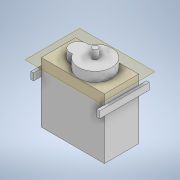
# Autodesk Inventor part: Part1
Saved by Autodesk Inventor 2021.1 (Build 251245010, 245A)
## iProperties
Created: 2023-07-02
Part Number: Part1
Material: Generic
Document SubType Name: Modeling
Designer: Drake
Density: 1 g/cm^3
Appearance: Default
Author: Drake
Autodesk Inventor part; units mm, degrees
sketch "Sketch1" plane through (0, 0, 0) normal (0, 1, 0) x (-1, 0, 0)
  line L0 (11.5, -6.25) -> (-11.5, -6.25)
  line L1 (-11.5, -6.25) -> (-11.5, 6.25)
  line L2 (-11.5, 6.25) -> (11.5, 6.25)
  line L3 (11.5, 6.25) -> (11.5, -6.25)
  line L4 (11.5, -6.25) -> (-11.5, 6.25) construction
  line L5 (-11.5, -6.25) -> (11.5, 6.25) construction
  point P0 (0, 0)
  dimension "d0" = 23
  dimension "d1" = 12.5
  constraints: 12 end point, 2 midpoint, 2 parallel, 1 horizontal, 1 perpendicular
  measures "d0" distance of L1.end L2.end
  measures "d1" distance of L2.end L0.start
extrude "Extrusion1" add sketch "Sketch1" along normal mid plane 22
ref_plane "Work Plane3" through (-11.5, 0, 0) normal (1, 0, 0) x (0, 1, 0)
ref_plane "Work Plane2" through (11.5, 0, 0) normal (1, 0, 0) x (0, 1, 0)
ref_plane "Work Plane4" through (0, 5, 0) normal (0, 1, 0) x (-1, 0, 0)
ref_plane "Work Plane5" through (0, 0, 6.25) normal (0, 0, 1) x (1, 0, 0)
sketch "Sketch2" plane through (11.5, -11, -6.25) normal (1, 0, 0) x (0, 0, -1)
  line L0 (0, 0) -> (-12.5, 0) projected
  line L1 (-12.5, 0) -> (-12.5, 16)
  line L2 (-12.5, 0) -> (-12.5, 22) projected
  line L3 (-12.5, 16) -> (-15.3, 16)
  line L4 (-15.3, 16) -> (-15.3, 18.5)
  line L5 (-15.3, 18.5) -> (0, 18.5)
  line L6 (0, 18.5) -> (2.8, 18.5)
  line L7 (2.8, 18.5) -> (2.8, 16)
  line L8 (2.8, 16) -> (-12.5, 16)
  point P0 (-6.25, 11)
  dimension "d8" = 16
  dimension "d9" = 2.8
  dimension "d10" = 2.5
  dimension "d11" = 2.8
  constraints: 14 end point, 4 perpendicular, 3 point on line, 1 horizontal
  measures "d8" distance of L0.end L1.end
  measures "d9" distance of L1.end L3.end
  measures "d10" distance of L3.end L4.end
  measures "d11" distance of L5.end L6.end
extrude "Extrusion2" add sketch "Sketch2" along normal blind 1
mirror "Mirror1" about plane through (0, 0, 0) normal (1, 0, 0) of "Extrusion2"
ref_plane "Work Plane6" through (0, 11, 0) normal (0, 1, 0) x (-1, 0, 0)
sketch "Sketch3" plane through (0, 11, 0) normal (0, 1, 0) x (-1, 0, 0)
  line L0 (-12.5008, 0) -> (-1.9008, 0)
  arc A0 (3.4585, 2.9134) -> (3.4585, -2.9134) centre (-1.9008, 0) ccw
  circle A1 centre (-1.9008, 0) radius 1
  arc A2 (3.4585, -2.9134) -> (3.4585, 2.9134) centre (4.1992, 0) ccw
  point P0 (0, 0)
  dimension "d15" = 10.6
  dimension "d16" = 12.2
  dimension "d17" = 2
  constraints: 5 point on circle, 3 centre point, 2 coincident, 2 end point, 1 horizontal
  measures "d15" distance of L0.start L0.end
  measures "d16" diameter of A0
  measures "d17" diameter of A1
extrude "Extrusion3" add sketch "Sketch3" along normal blind 3.5
sketch "Sketch4" plane through (0, 14.5, 0) normal (0, 1, 0) x (1, 0, 0)
  circle A0 centre (1.9008, 0) radius 1 projected
  circle A1 centre (1.9008, 0) radius 2
  point P0 (0, 0)
  dimension "d20" = 4
  constraints: 1 centre point, 1 coincident
  measures "d20" diameter of A1
extrude "Extrusion4" add sketch "Sketch4" along normal blind 3.2 contours A0
body "Solid1"
